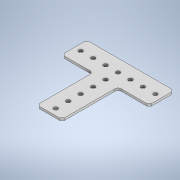
# Autodesk Inventor part: TGusset Versa
Saved by Autodesk Inventor 2020 (Build 240168000, 168)
## iProperties
Created: 2020-01-14
Part Number: TGusset Versa
Material: Generic
Document SubType Name: Modeling
Designer: aidan
Density: 1 g/cm^3
Appearance: Default
Author: aidan
Autodesk Inventor part; units mm, degrees
ref_plane "YZ Plane" through (0, 0, 0) normal (1, 0, 0) x (0, 1, 0)
ref_plane "XZ Plane" through (0, 0, 0) normal (0, 1, 0) x (-1, 0, 0)
ref_plane "XY Plane" through (0, 0, 0) normal (0, 0, 1) x (1, 0, 0)
sketch "Sketch1" plane through (0, 0, 0) normal (0, 1, 0) x (-1, 0, 0)
  line L0 (69.0976, -38.7621) -> (24.6476, -38.7621)
  line L1 (69.0976, -13.3621) -> (69.0976, -38.7621)
  line L2 (24.6476, -38.7621) -> (41.922, -38.7621)
  line L3 (37.3476, 43.7879) -> (24.6476, 43.7879)
  line L4 (69.0976, -13.3621) -> (37.3476, -13.3621)
  line L5 (37.3476, -13.3621) -> (37.3476, 43.7879)
  line L6 (-19.8024, -38.7621) -> (24.6476, -38.7621)
  line L7 (-19.8024, -13.3621) -> (-19.8024, -38.7621)
  line L8 (24.6476, -38.7621) -> (7.3732, -38.7621)
  line L9 (11.9476, 43.7879) -> (24.6476, 43.7879)
  line L10 (-19.8024, -13.3621) -> (11.9476, -13.3621)
  line L11 (11.9476, -13.3621) -> (11.9476, 43.7879)
  point P0 (0, 0)
  dimension "d0" = 44.45
  dimension "d1" = 12.7
  dimension "d2" = 25.4
  dimension "d3" = 82.55
  constraints: 24 end point, 3 horizontal, 1 parallel, 1 perpendicular
  measures "d0" distance of L0.start L0.end
  measures "d1" distance of L3.start L3.end
  measures "d2" distance of L1.start L0.start
  measures "d3" distance between parallel lines of L3 L0
extrude "Extrusion1" add sketch "Sketch1" along normal blind 2.286
sketch "Sketch2" plane through (0, 2.286, 0) normal (0, 1, 0) x (1, 0, 0)
  circle A0 centre (-24.6476, 26.0621) radius 2.0828
  line L0 (19.8024, 38.7621) -> (-69.0976, 38.7621) projected
  line L1 (19.8024, 13.3621) -> (19.8024, 38.7621) projected
  point P0 (0, 0)
  dimension "d6" = 4.1656
  dimension "d7" = 12.7
  dimension "d8" = 44.45
  constraints: 1 centre point
  measures "d6" diameter of A0
  measures "d7" distance from line of L0 A0.centre
  measures "d8" distance from line of L1 A0.centre
extrude "Extrusion2" cut sketch "Sketch2" against normal blind 2.286
pattern_linear "Rectangular Pattern1" count 4 spacing 12.7 along (1, 0, 0) count 4 spacing 12.7 along (-1, 0, 0) of "Extrusion2"
pattern_linear "Rectangular Pattern2" count 6 spacing 12.7 along (0, 0, 1) of "Extrusion2"
chamfer "Chamfer1" distance 2.54 angle 45 6 edges at (-69.0976, 1.143, -13.3621) (-37.3476, 1.143, 43.7879) (-11.9476, 1.143, 43.7879) (19.8024, 1.143, -13.3621) (19.8024, 1.143, -38.7621) (-69.0976, 1.143, -38.7621)
fillet "Fillet1" radius 3.175 2 edges at (-37.3476, 1.143, -13.3621) (-11.9476, 1.143, -13.3621)
body "Solid1"
